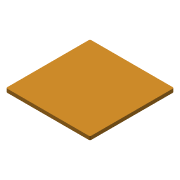
# Autodesk Inventor part: 3136 1094 58
Saved by Autodesk Inventor 2022 Beta2 (Build 260130000, 130) ContinuousBuild 0
## iProperties
Shininess: 64.0
Length Units: 11269
Angle Units: 11279
Time Units: 11290
Mass Units: 11283
Length Display Precision: 3
Angle Display Precision: 2
Compacted: True
Part Number: 3136 1094 58
Document SubType Name: Modeling
Created: 2003-04-13
Material: Steel, Mild
Designer: Uffe Bak
Density: 7.86 g/cm^3
Appearance: Brokk-Gul
Density: 0.0
Volumn: 0.0
Area: 0.0
PropertySet Name: Model Information
Control State: 0
Master: False
Checked Out: False
Author: Uffe Bak
Autodesk Inventor part; units mm, degrees
ref_plane "YZ Plane" through (0, 0, 0) normal (1, 0, 0) x (0, 1, 0)
ref_plane "XZ Plane" through (0, 0, 0) normal (0, 1, 0) x (-1, 0, 0)
ref_plane "XY Plane" through (0, 0, 0) normal (0, 0, 1) x (1, 0, 0)
sketch "Sketch1" plane through (0, 0, 0) normal (0, 0, 1) x (1, 0, 0)
  line L0 (35, 34) -> (35, -34)
  line L1 (34, -35) -> (-34, -35)
  line L2 (-35, -34) -> (-35, 34)
  line L3 (-34, 35) -> (34, 35)
  arc A0 (-34, 35) -> (-35, 34) centre (-34, 34) ccw
  arc A1 (35, 34) -> (34, 35) centre (34, 34) ccw
  arc A2 (34, -35) -> (35, -34) centre (34, -34) ccw
  arc A3 (-35, -34) -> (-34, -35) centre (-34, -34) ccw
  point P0 (0, 0)
  point P1 (0, 0)
  point P2 (35, 35)
  point P3 (35, -35)
  point P4 (-35, -35)
  point P5 (-35, 35)
  dimension "d0" = 70
  dimension "d1" = 1
  constraints: 8 end point, 8 point on circle, 8 point on line, 8 tangent, 4 centre point, 3 equal radius, 1 coincident, 7 other
  measures "d0" distance of point (-35, 35) point (35, 35)
  measures "d1" radius of A0
extrude "Extrusion1" add sketch "Sketch1" along normal blind 3
body "Solid1"
